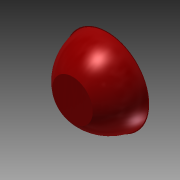
# Autodesk Inventor part: Pièce2
Saved by Autodesk Inventor 2015 (Build 190159000, 159)
## iProperties
Created: 2019-02-09
Part Number: Pièce2
Material: Générique
Document SubType Name: Modeling
Designer: Naly jérémie
Density: 1 g/cm^3
Appearance: Rouge
Author: Naly jérémie
Autodesk Inventor part; units mm, degrees
ref_plane "YZ Plane" through (0, 0, 0) normal (1, 0, 0) x (0, 1, 0)
ref_plane "XZ Plane" through (0, 0, 0) normal (0, 1, 0) x (-1, 0, 0)
ref_plane "XY Plane" through (0, 0, 0) normal (0, 0, 1) x (1, 0, 0)
sketch "Esquisse1" plane through (0, 0, 0) normal (0, 0, 1) x (1, 0, 0)
  line L0 (0, 0) -> (70, 0)
  line L1 (1.127, 4.5) -> (70, 4.5)
  arc A0 (70, 4.5) -> (138.2953, 119.6825) centre (-28.041, 140.47) ccw
  arc A1 (145.1172, 119.6184) -> (138.2953, 119.6825) centre (141.66, 114.7284) ccw
  line L2 (145.1172, 119.6184) -> (141.9857, 119.6184)
  arc A2 (70, 0) -> (141.9857, 119.6184) centre (-28.041, 140.47) ccw
  line L3 (1.127, 4.5) -> (0, 4.5)
  line L4 (0, 4.5) -> (0, 0)
  line L5 (0, 137.8568) -> (0, -38.4638)
  dimension "d0" = 70
  dimension "d3" = 4.5
  dimension "d4" = 70
  constraints: 12 end point, 7 point on circle, 3 centre point, 3 horizontal, 2 vertical, 1 concentric, 1 perpendicular, 1 point on line
  measures "d0" distance of L0.start L0.end
  measures "d3" distance of L3.end L0.start
  measures "d4" distance of L1.end L3.end
revolve "Révolution1" add sketch "Esquisse1" angle 360 about axis through (0, 137.8568, 0) along (0, -1, 0)
